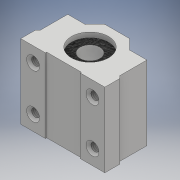
# Autodesk Inventor part: cojinete lineal
Saved by Autodesk Inventor 2018 (Build 220112000, 112)
## iProperties
Created: 2019-05-16
Part Number: cojinete lineal
Material: Generic
Document SubType Name: Modeling
Designer: JLVega003
Density: 1 g/cm^3
Appearance: Default
Author: JLVega003
Autodesk Inventor part; units mm, degrees
ref_plane "YZ Plane" through (0, 0, 0) normal (1, 0, 0) x (0, 1, 0)
ref_plane "XZ Plane" through (0, 0, 0) normal (0, 1, 0) x (-1, 0, 0)
ref_plane "XY Plane" through (0, 0, 0) normal (0, 0, 1) x (1, 0, 0)
sketch "Sketch1" plane through (0, 0, 0) normal (0, 0, 1) x (1, 0, 0)
  line L0 (-17, 0) -> (-7, 0)
  line L1 (-7, 0) -> (-7, 0.5)
  line L2 (-7, 0.5) -> (7, 0.5)
  line L3 (7, 0.5) -> (7, 0)
  line L4 (7, 0) -> (17, 0)
  line L5 (17, 0) -> (17, 6)
  line L6 (17, 6) -> (16, 7)
  line L7 (16, 7) -> (16, 18)
  line L8 (16, 18) -> (9, 18)
  line L9 (9, 18) -> (5, 22)
  line L10 (5, 22) -> (-5, 22)
  line L11 (-5, 22) -> (-9, 18)
  line L12 (-9, 18) -> (-16, 18)
  line L13 (-16, 18) -> (-16, 7)
  line L14 (-16, 7) -> (-17, 6)
  line L15 (-17, 6) -> (-17, 0)
  line L16 (-23.8, 0) -> (23.8, 0) construction
  line L17 (0, -4.4) -> (0, 26.4) construction
  circle A0 centre (0, 11) radius 4
  line L18 (-7, 0.5) -> (-7, 20) construction
  point P0 (0, 0)
  point P1 (0, 22)
  point P2 (0, 0.5)
  dimension "d0" = 34
  dimension "d1" = 14
  dimension "d2" = 6
  dimension "d3" = 18
  dimension "d5" = 11
  dimension "d6" = 8
  dimension "d7" = 0.5
  dimension "d8" = 45
  dimension "d9" = 45
  dimension "d10" = 1
  dimension "d11" = 1
  dimension "d12" = 6
  dimension "d13" = 45
  dimension "d33" = 22
  constraints: 34 end point, 7 perpendicular, 4 midpoint, 4 parallel, 4 point on line, 3 collinear, 1 centre point, 1 horizontal, 1 vertical
  measures "d0" distance between parallel lines of L5 L15
  measures "d1" distance between parallel lines of L3 L1
  measures "d2" distance of L14.end L0.start
  measures "d3" distance between parallel lines of L12 L16
  measures "d5" distance from line of A0.centre L0
  measures "d6" diameter of A0
  measures "d7" distance between parallel lines of L0 L2
  measures "d8" angle of L14 L15
  measures "d9" angle of L5 L6
  measures "d10" distance between parallel lines of L13 L15
  measures "d11" distance between parallel lines of L5 L7
  measures "d12" distance of L4.end L5.end
  measures "d13" angle of L8 L9
  measures "d33" distance between parallel lines of L16 L10
extrude "Extrusion1" add sketch "Sketch1" along normal mid plane 30
sketch "Sketch2" plane through (0, 0, -15) normal (0, 0, -1) x (-1, 0, 0)
  circle A0 centre (0, 11) radius 4 projected
  circle A1 centre (0, 11) radius 7.5
  point P0 (0, 0)
  dimension "d17" = 15
  constraints: 1 centre point, 1 coincident
  measures "d17" diameter of A1
extrude "Extrusion2" cut sketch "Sketch2" against normal blind 2
mirror "Mirror1" about plane through (0, 0, 0) normal (0, 0, 1) of "Extrusion2"
sketch "Sketch3" plane through (7, 0, 15) normal (0, -1, 0) x (1, 0, 0)
  line L0 (10, -30) -> (10, 0) construction
  line L1 (0, 0) -> (10, 0) construction
  line L2 (0, -30) -> (0, 0) construction
  line L3 (10, -30) -> (0, -30) construction
  line L4 (-14, -30) -> (-14, 0) construction
  line L5 (-24, 0) -> (-14, 0) construction
  line L6 (-24, 0) -> (-24, -30) construction
  line L7 (-14, -30) -> (-24, -30) construction
  line L8 (5, -6) -> (-19, -6) construction
  line L9 (-19, -6) -> (-19, -24) construction
  line L10 (-19, -24) -> (5, -24) construction
  line L11 (5, -24) -> (5, -6) construction
  line L12 (5, -6) -> (-19, -24) construction
  line L13 (-19, -6) -> (5, -24) construction
  point P0 (-7, -15)
  dimension "d21" = 18
  dimension "d29" = 24
  constraints: 12 end point, 4 coincident, 2 midpoint, 2 parallel, 1 horizontal, 1 perpendicular
  measures "d21" distance between parallel lines of L8 L10
  measures "d29" distance between parallel lines of L9 L11
hole "Hole1" at (12, 0, -9) at (-12, 0, -9) at (12, 0, 9) at (-12, 0, 9) direction (0, 1, 0) diameter 3.242 end through all thread size "M4x0.7" class "6H" standard "ISO Metric profile"
chamfer "Chamfer1" distance 1 angle 45 4 edges at (12, 0, -7.379) (-12, 0, -7.379) (-12, 0, 10.621) (12, 0, 10.621)
ref_plane "Work Plane1" through (0, 0, 0) normal (0, 0, 1) x (1, 0, 0)
equation "\"d9\" = d8"
equation "\"d11\" = d10"
equation "\"d12\" = d2"
body "Solid1"
